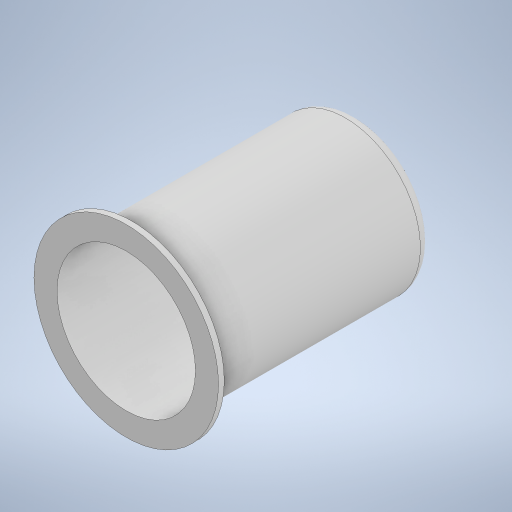
# Autodesk Inventor part: насадка для катпака
Saved by Autodesk Inventor 2023.1 (Build 271208000, 208)
## iProperties
Created: 2023-06-20
Part Number: насадка для катпака
Material: Типовые
Document SubType Name: Modeling
Designer: User
Density: 1 g/cm^3
Appearance: По умолчанию
Author: User
Autodesk Inventor part; units mm, degrees
ref_plane "YZ Plane" through (0, 0, 0) normal (1, 0, 0) x (0, 1, 0)
ref_plane "XZ Plane" through (0, 0, 0) normal (0, 1, 0) x (-1, 0, 0)
ref_plane "XY Plane" through (0, 0, 0) normal (0, 0, 1) x (1, 0, 0)
sketch "Эскиз1" plane through (0, 0, 0) normal (0, 0, 1) x (1, 0, 0)
  circle A0 centre (0, 0) radius 13
  circle A1 centre (0, 0) radius 12
  dimension "d0" = 26
  dimension "d1" = 24
  constraints: 2 centre point, 2 coincident
  measures "d0" diameter of A0
  measures "d1" diameter of A1
extrude "Выдавливание1" add sketch "Эскиз1" along normal blind 38
sketch "Эскиз2" plane through (0, 0, 38) normal (0, 0, 1) x (1, 0, 0)
  circle A0 centre (0, 0) radius 16
  circle A1 centre (0, 0) radius 12
  dimension "d4" = 32
  dimension "d5" = 24
  constraints: 2 centre point, 2 coincident
  measures "d4" diameter of A0
  measures "d5" diameter of A1
extrude "Выдавливание2" add sketch "Эскиз2" along normal blind 1
sketch "Эскиз3" plane through (0, 0, 0) normal (0, 0, -1) x (-1, 0, 0)
  circle A0 centre (0, 0) radius 13 projected
extrude "Выдавливание3" add sketch "Эскиз3" along normal blind 1
fillet "Сопряжение1" radius 2 1 edges at (-12, 0, 0)
fillet "Сопряжение2" radius 2 1 edges at (13, 0, -1)
sketch "Эскиз4" plane through (0, 0, -1) normal (0, 0, -1) x (-1, 0, 0)
  line L0 (-2.25, -2.25) -> (2.25, -2.25)
  line L1 (2.25, -2.25) -> (2.25, 2.25)
  line L2 (2.25, 2.25) -> (-2.25, 2.25)
  line L3 (-2.25, 2.25) -> (-2.25, -2.25)
  line L4 (22.4, 0) -> (-22.4, 0) projected
  line L5 (0, -22.4) -> (0, 22.4) projected
  point P0 (0, 0)
  dimension "d12" = 4.5
  dimension "d13" = 4.5
  constraints: 8 end point, 2 parallel, 1 horizontal, 1 perpendicular, 2 other
  measures "d12" distance between parallel lines of L2 L0
  measures "d13" distance between parallel lines of L1 L3
extrude "Выдавливание4" cut sketch "Эскиз4" against normal blind 1
sketch "Эскиз5" plane through (0, 0, -1) normal (0, 0, -1) x (-1, 0, 0)
  line L0 (-2.25, 2.25) -> (2.25, 2.25) projected
  line L1 (-2.25, -2.25) -> (-2.25, 2.25) projected
  line L2 (2.25, -2.25) -> (-2.25, -2.25) projected
  line L3 (2.25, 2.25) -> (2.25, -2.25) projected
  line L4 (-3.25, -3.25) -> (3.25, -3.25)
  line L5 (3.25, -3.25) -> (3.25, 3.25)
  line L6 (3.25, 3.25) -> (-3.25, 3.25)
  line L7 (-3.25, 3.25) -> (-3.25, -3.25)
  point P0 (0, 0)
  dimension "d16" = 1
  dimension "d17" = 1
  dimension "d18" = 1
  dimension "d19" = 1
  constraints: 8 end point, 2 parallel, 1 horizontal, 1 perpendicular
  measures "d16" distance between parallel lines of L2 L4
  measures "d17" distance between parallel lines of L6 L0
  measures "d18" distance between parallel lines of L7 L1
  measures "d19" distance between parallel lines of L5 L3
extrude "Выдавливание5" add sketch "Эскиз5" along normal blind 5
